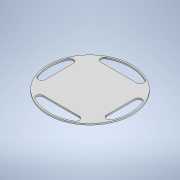
# Autodesk Inventor part: InnerCap
Saved by Autodesk Inventor 2021 (Build 250183000, 183)
## iProperties
Created: 2022-01-13
Part Number: InnerCap
Material: Типовые
Document SubType Name: Modeling
Designer: Maxim
Density: 1 g/cm^3
Appearance: По умолчанию
Author: Maxim
Autodesk Inventor part; units mm, degrees
ref_plane "YZ Plane" through (0, 0, 0) normal (1, 0, 0) x (0, 1, 0)
ref_plane "XZ Plane" through (0, 0, 0) normal (0, 1, 0) x (-1, 0, 0)
ref_plane "XY Plane" through (0, 0, 0) normal (0, 0, 1) x (1, 0, 0)
sketch "Эскиз1" plane through (0, 0, 0) normal (0, 1, 0) x (-1, 0, 0)
  circle A0 centre (0, 0) radius 58.5
  line L0 (40, -37.5) -> (-40, -37.5) construction
  line L1 (-40, -37.5) -> (-40, 37.5) construction
  line L2 (-40, 37.5) -> (40, 37.5) construction
  line L3 (40, 37.5) -> (40, -37.5) construction
  line L4 (40, -37.5) -> (-40, 37.5) construction
  line L5 (-40, -37.5) -> (40, 37.5) construction
  line L6 (-42.6779, -40.0106) -> (42.6779, -40.0106)
  line L7 (42.6779, -40.0106) -> (42.6779, 40.0106)
  line L8 (42.6779, 40.0106) -> (-42.6779, 40.0106)
  line L9 (-42.6779, 40.0106) -> (-42.6779, -40.0106)
  line L10 (-42.6779, -40.0106) -> (42.6779, 40.0106) construction
  line L11 (42.6779, -40.0106) -> (-42.6779, 40.0106) construction
  arc A1 (25.026, 40.0106) -> (27.4557, 49.3805) centre (25.026, 45.0106) ccw
  circle A2 centre (0, 0) radius 56.5
  arc A3 (-27.4557, 49.3805) -> (-25.026, 40.0106) centre (-25.026, 45.0106) ccw
  arc A4 (52.3069, 21.3599) -> (42.6779, 19.4696) centre (47.6779, 19.4696) ccw
  arc A5 (42.6779, -19.4696) -> (52.3069, -21.3599) centre (47.6779, -19.4696) ccw
  arc A6 (27.4557, -49.3805) -> (25.026, -40.0106) centre (25.026, -45.0106) ccw
  arc A7 (-25.026, -40.0106) -> (-27.4557, -49.3805) centre (-25.026, -45.0106) ccw
  arc A8 (-52.3069, -21.3599) -> (-42.6779, -19.4696) centre (-47.6779, -19.4696) ccw
  arc A9 (-42.6779, 19.4696) -> (-52.3069, 21.3599) centre (-47.6779, 19.4696) ccw
  dimension "d0" = 117
  dimension "d3" = 113
  dimension "d1" = 80
  dimension "d2" = 75
  dimension "d4" = 10
  dimension "d5" = 10
  dimension "d6" = 10
  dimension "d7" = 10
  dimension "d8" = 10
  dimension "d9" = 10
  dimension "d10" = 10
  dimension "d11" = 10
  constraints: 24 end point, 16 point on circle, 9 point on line, 8 centre point, 8 tangent, 4 midpoint, 4 parallel, 2 coincident, 2 horizontal, 2 perpendicular, 21 other
  measures "d1" distance of L1.end L2.end
  measures "d2" distance of L0.end L1.end
  measures "d4" diameter of A1
  measures "d5" diameter of A3
  measures "d6" diameter of A4
  measures "d7" diameter of A5
  measures "d8" diameter of A6
  measures "d9" diameter of A7
  measures "d10" diameter of A8
  measures "d11" diameter of A9
extrude "Выдавливание1" add sketch "Эскиз1" along normal blind 2 contours A0 L7 A2 | L8 A2 A0 | L7 A2 L8 | A0 L6 A2 | L6 A2 L7 | L9 A2 A0 | L8 A2 L9 | A2 A4 L7 | L7 A2 L6 L9 L8 | L8 A1 A2 | L9 A2 L6 | A2 A6 L6 | L7 A5 A2 | A2 A3 L8 | L9 A9 A2 | L6 A7 A2 | A2 A8 L9
